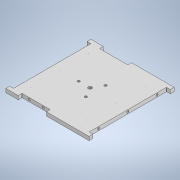
# Autodesk Inventor part: baza
Saved by Autodesk Inventor 2020 (Build 240168000, 168)
## iProperties
Created: 2020-08-17
Part Number: baza
Material: Generic
Document SubType Name: Modeling
Designer: Hesekiel
Density: 1 g/cm^3
Appearance: Default
Author: Hesekiel
Autodesk Inventor part; units mm, degrees
ref_plane "YZ Plane" through (0, 0, 0) normal (1, 0, 0) x (0, 1, 0)
ref_plane "XZ Plane" through (0, 0, 0) normal (0, 1, 0) x (-1, 0, 0)
ref_plane "XY Plane" through (0, 0, 0) normal (0, 0, 1) x (1, 0, 0)
sketch "Sketch1" plane through (0, 0, 0) normal (0, 1, 0) x (-1, 0, 0)
  line L0 (-50, 112.5) -> (50, 112.5)
  line L1 (50, 112.5) -> (50, -112.5)
  line L2 (50, -112.5) -> (-50, -112.5)
  line L3 (-50, -112.5) -> (-50, 112.5)
  line L4 (-50, 112.5) -> (50, -112.5) construction
  line L5 (50, 112.5) -> (-50, -112.5) construction
  line L6 (-37.5, -102.5) -> (37.5, -102.5)
  line L7 (37.5, -102.5) -> (37.5, 102.5)
  line L8 (37.5, 102.5) -> (-37.5, 102.5)
  line L9 (-37.5, 102.5) -> (-37.5, -102.5)
  line L10 (-37.5, -102.5) -> (37.5, 102.5) construction
  line L11 (37.5, -102.5) -> (-37.5, 102.5) construction
  line L12 (37.5, 112.5) -> (37.5, -112.5)
  line L13 (-37.5, 112.5) -> (-37.5, -112.5)
  line L14 (-50, -112.5) -> (-150, -112.5)
  line L15 (-150, 112.5) -> (-50, 112.5)
  line L16 (-50, 112.5) -> (-50, -112.5)
  line L17 (-150, -112.5) -> (-140, -112.5)
  line L18 (-140, -112.5) -> (-140, 112.5)
  line L19 (-150, -112.5) -> (-150, -102.5)
  line L20 (-150, -102.5) -> (-140, -102.5)
  line L21 (-140, 112.5) -> (-140, 102.5)
  line L22 (-140, 102.5) -> (-150, 102.5)
  line L23 (50, 112.5) -> (70, 112.5)
  line L24 (70, -112.5) -> (50, -112.5)
  line L25 (50, -112.5) -> (50, 112.5)
  line L26 (70, -112.5) -> (70, -102.5)
  line L27 (70, 112.5) -> (70, 102.5)
  line L28 (70, -102.5) -> (60, -102.5)
  line L29 (60, -102.5) -> (60, 102.5)
  line L30 (60, 102.5) -> (70, 102.5)
  line L31 (-150, 102.5) -> (-150, 112.5)
  point P0 (0, 0)
  dimension "d0" = 100
  dimension "d2" = 75
  dimension "d3" = 205
  dimension "d49" = 100
  dimension "d50" = 10
  dimension "d51" = 10
  dimension "d52" = 10
  constraints: 64 end point, 11 point on line, 7 parallel, 5 horizontal, 5 perpendicular, 4 midpoint, 1 vertical
  measures "d0" distance of L1.end L2.end
  measures "d2" distance of L8.end L7.end
  measures "d3" distance of L7.end L6.end
  measures "d49" distance of L15.start L15.end
  measures "d50" distance of L14.end L17.end
  measures "d51" distance of L14.end L19.end
  measures "d52" distance of L18.end L21.end
extrude "Extrusion1" add sketch "Sketch1" along normal blind 10 contours L0 L13 L9 L2 L3 | L3 L14 L18 L15 | L18 L22 L31 L15 | L0 L1 L2 L12 L7 | L8 L7 L6 L9 | L14 L19 L20 L18 | L23 L27 L30 L29 L28 L26 L24 L1
sketch "Sketch2" plane through (-37.5, 0, 102.5) normal (0, 0, 1) x (1, 0, 0)
  line L0 (0, 0) -> (75, 0) projected
  line L1 (75, 0) -> (75, 10) projected
  line L2 (0, 10) -> (75, 10) projected
  line L3 (0, 0) -> (0, 10) projected
  line L4 (37.5, 0) -> (37.5, 10)
  line L5 (75, 10) -> (0, 10) projected
  line L6 (37.5, 5) -> (0, 5)
  line L7 (0, 0) -> (0, 10) projected
  line L8 (37.5, 5) -> (75, 5)
  line L9 (75, 0) -> (75, 10) projected
  circle A0 centre (18.75, 5) radius 3
  circle A1 centre (56.25, 5) radius 3
  dimension "d6" = 6
  dimension "d7" = 6
  constraints: 6 end point, 6 midpoint, 2 centre point
  measures "d6" diameter of A0
  measures "d7" diameter of A1
extrude "Extrusion2" cut sketch "Sketch2" against normal blind 20 contours A0 L6 | L6 A0 | A1 L8 | L8 A1
thread "Thread1" size "M6x1" class "6H" standard "ANSI Metric M Profile" full length
thread "Thread2" size "M6x1" class "6H" standard "ANSI Metric M Profile" full length
sketch "Sketch3" plane through (37.5, 0, -102.5) normal (0, 0, -1) x (-1, 0, 0)
  circle A0 centre (18.75, 5) radius 3 projected
  circle A1 centre (56.25, 5) radius 3 projected
  point P0 (37.5, 0)
extrude "Extrusion3" cut sketch "Sketch3" against normal blind 20
thread "Thread3" size "M6x1" class "6H" standard "ANSI Metric M Profile" full length
thread "Thread4" size "M6x1" class "6H" standard "ANSI Metric M Profile" full length
sketch "Sketch4" plane through (-18.75, 5, 82.5) normal (0, 0, 1) x (1, 0, 0)
  point P0 (0, 0)
hole "Hole1" at (-18.75, 5, 82.5) direction (0, 0, -1) diameter 4.917 depth 3 tip angle 120 thread size "M6x1" class "6H" standard "ISO Metric profile"
sketch "Sketch5" plane through (18.75, 5, 82.5) normal (0, 0, 1) x (1, 0, 0)
  point P0 (0, 0)
hole "Hole3" at (18.75, 5, 82.5) direction (0, 0, -1) diameter 4.917 depth 3 tip angle 120 thread size "M6x1" class "6H" standard "ISO Metric profile"
sketch "Sketch6" plane through (18.75, 5, -82.5) normal (0, 0, -1) x (-1, 0, 0)
  point P0 (0, 0)
hole "Hole5" at (18.75, 5, -82.5) direction (0, 0, 1) diameter 4.917 depth 3 tip angle 120 thread size "M6x1" class "6H" standard "ISO Metric profile"
sketch "Sketch7" plane through (-18.75, 5, -82.5) normal (0, 0, -1) x (-1, 0, 0)
  point P0 (0, 0)
hole "Hole7" at (-18.75, 5, -82.5) direction (0, 0, 1) diameter 4.917 depth 3 tip angle 120 thread size "M6x1" class "6H" standard "ISO Metric profile"
fillet "Fillet1" radius 1 6 edges at (-37.5, 5, 102.5) (37.5, 5, 102.5) (-37.5, 5, -102.5) (37.5, 5, -102.5) (140, 5, -102.5) (140, 5, 102.5)
sketch "Sketch8" plane through (140, 0, 101.5) normal (1, 0, 0) x (0, 0, -1)
  line L0 (0, 0) -> (0, 10) projected
  line L1 (0, 0) -> (203, 0) projected
  line L2 (203, 10) -> (203, 0) projected
  line L3 (0, 10) -> (203, 10) projected
  line L4 (214, 10) -> (-11, 10) projected
  circle A0 centre (101.5, 5) radius 3
  line L5 (203, 10) -> (203, 0) projected
  circle A1 centre (179, 5) radius 3
  circle A2 centre (24, 5) radius 3
  line L6 (-1, 0) -> (-1, 10) projected
  line L7 (-1, 5) -> (24, 5)
  line L8 (24, 5) -> (101.5, 5)
  line L9 (204, 0) -> (214, 0) projected
  line L10 (214, 0) -> (214, 10) projected
  line L11 (204, 10) -> (214, 10) projected
  line L12 (204, 0) -> (204, 10) projected
  line L13 (214, 0) -> (214, 10) projected
  line L14 (214, 10) -> (204, 10) projected
  line L15 (204, 0) -> (204, 10) projected
  line L16 (101.5, 5) -> (179, 5)
  point P0 (101.5, 0)
  dimension "d54" = 6
  dimension "d57" = 6
  dimension "d59" = 6
  dimension "d130" = 25
  dimension "d131" = 77.5
  constraints: 6 end point, 3 centre point, 2 perpendicular, 1 horizontal, 1 midpoint
  measures "d54" diameter of A0
  measures "d57" diameter of A1
  measures "d59" diameter of A2
  measures "d130" distance of L7.start L7.end
  measures "d131" distance of L8.end L16.end
extrude "Extrusion4" cut sketch "Sketch8" against normal blind 30 contours L16 L8 A0 | A0 L8 L16 | A1 | L8 L7 A2 | A2 L7 L8
thread "Thread5" size "M6x1" class "6H" standard "ANSI Metric M Profile" full length
thread "Thread6" size "M6x1" class "6H" standard "ANSI Metric M Profile" full length
thread "Thread7" size "M6x1" class "6H" standard "ANSI Metric M Profile" full length
sketch "Sketch12" plane through (-60, 0, -102.5) normal (-1, 0, 0) x (0, 0, 1)
  circle A0 centre (25, 5) radius 3 projected
  circle A1 centre (102.5, 5) radius 3 projected
  circle A2 centre (180, 5) radius 3 projected
  line L0 (204, 0) -> (204, 10) projected
  line L1 (204, 0) -> (1, 0) projected
  line L2 (1, 10) -> (1, 0) projected
  line L3 (204, 10) -> (1, 10) projected
  point P0 (102.5, 0)
extrude "Extrusion5" cut sketch "Sketch12" against normal blind 20 contours A0 | A1 | A2
thread "Thread8" size "M6x1" class "6H" standard "ANSI Metric M Profile" full length
thread "Thread9" size "M6x1" class "6H" standard "ANSI Metric M Profile" full length
thread "Thread10" size "M6x1" class "6H" standard "ANSI Metric M Profile" full length
sketch "Sketch9" plane through (110, 5, 77.5) normal (1, 0, 0) x (0, 0, -1)
  point P0 (-0.375, 0)
sketch "Sketch10" plane through (110, 5, 0) normal (1, 0, 0) x (0, 0, -1)
  point P0 (0, 0)
sketch "Sketch11" plane through (110, 5, -77.5) normal (1, 0, 0) x (0, 0, -1)
  point P0 (0.375, 0)
sketch "Sketch13" plane through (-40, 5, -77.5) normal (-1, 0, 0) x (0, 0, 1)
  point P0 (0.625, 0)
sketch "Sketch14" plane through (-40, 5, 0) normal (-1, 0, 0) x (0, 0, 1)
  point P0 (0, 0)
sketch "Sketch15" plane through (-40, 5, 77.5) normal (-1, 0, 0) x (0, 0, 1)
  point P0 (0.375, 0)
sketch "Sketch16" plane through (110, 5, 77.5) normal (1, 0, 0) x (0, 0, -1)
  point P0 (0, 0)
hole "Hole20" at (110, 5, 77.5) direction (-1, 0, 0) diameter 4.917 depth 3 tip angle 120 thread size "M6x1" class "6H" standard "ISO Metric profile"
sketch "Sketch17" plane through (110, 5, 0) normal (1, 0, 0) x (0, 0, -1)
  point P0 (0, 0)
hole "Hole22" at (110, 5, 0) direction (-1, 0, 0) diameter 4.917 depth 3 tip angle 120 thread size "M6x1" class "6H" standard "ISO Metric profile"
sketch "Sketch18" plane through (110, 5, -77.5) normal (1, 0, 0) x (0, 0, -1)
  point P0 (0, 0)
hole "Hole24" at (110, 5, -77.5) direction (-1, 0, 0) diameter 4.917 depth 3 tip angle 120 thread size "M6x1" class "6H" standard "ISO Metric profile"
sketch "Sketch22" plane through (-40, 5, 77.5) normal (-1, 0, 0) x (0, 0, 1)
  point P0 (0, 0)
hole "Hole31" at (-40, 5, 77.5) direction (1, 0, 0) diameter 4.917 depth 8 tip angle 120 thread size "M6x1" class "6H" standard "ISO Metric profile"
sketch "Sketch23" plane through (-40, 5, 0) normal (-1, 0, 0) x (0, 0, 1)
  point P0 (0, 0)
hole "Hole33" at (-40, 5, 0) direction (1, 0, 0) diameter 4.917 depth 8 tip angle 120 thread size "M6x1" class "6H" standard "ISO Metric profile"
sketch "Sketch24" plane through (-40, 5, -77.5) normal (-1, 0, 0) x (0, 0, 1)
  point P0 (0, 0)
hole "Hole35" at (-40, 5, -77.5) direction (1, 0, 0) diameter 4.917 depth 8 tip angle 120 thread size "M6x1" class "6H" standard "ISO Metric profile"
sketch "Sketch25" plane through (0, 10, 0) normal (0, 1, 0) x (1, 0, 0)
  line L0 (-70, -112.5) -> (-37.5, -112.5) projected
  line L1 (-37.5, -112.5) -> (-37.5, -103.5) projected
  arc A0 (-36.5, -102.5) -> (-37.5, -103.5) centre (-36.5, -103.5) ccw projected
  line L2 (-36.5, -102.5) -> (36.5, -102.5) projected
  arc A1 (37.5, -103.5) -> (36.5, -102.5) centre (36.5, -103.5) ccw projected
  line L3 (37.5, -103.5) -> (37.5, -112.5) projected
  line L4 (37.5, -112.5) -> (150, -112.5) projected
  line L5 (150, -112.5) -> (150, -102.5) projected
  line L6 (150, -102.5) -> (141, -102.5) projected
  arc A2 (140, -101.5) -> (141, -102.5) centre (141, -101.5) ccw projected
  line L7 (140, -101.5) -> (140, 101.5) projected
  arc A3 (141, 102.5) -> (140, 101.5) centre (141, 101.5) ccw projected
  line L8 (141, 102.5) -> (150, 102.5) projected
  line L9 (150, 102.5) -> (150, 112.5) projected
  line L10 (150, 112.5) -> (37.5, 112.5) projected
  line L11 (37.5, 112.5) -> (37.5, 103.5) projected
  arc A4 (36.5, 102.5) -> (37.5, 103.5) centre (36.5, 103.5) ccw projected
  line L12 (36.5, 102.5) -> (-36.5, 102.5) projected
  arc A5 (-37.5, 103.5) -> (-36.5, 102.5) centre (-36.5, 103.5) ccw projected
  line L13 (-37.5, 103.5) -> (-37.5, 112.5) projected
  line L14 (-37.5, 112.5) -> (-70, 112.5) projected
  line L15 (-70, 112.5) -> (-70, 102.5) projected
  line L16 (-70, 102.5) -> (-60, 102.5) projected
  line L17 (-60, 102.5) -> (-60, -102.5) projected
  line L18 (-60, -102.5) -> (-70, -102.5) projected
  line L19 (-70, -102.5) -> (-70, -112.5) projected
  line L20 (140, -101.5) -> (140, 101.5) projected
  line L21 (140, 0) -> (-60, 0)
  line L22 (-60, -3) -> (-60, 3) projected
  line L23 (-70, -112.5) -> (-37.5, -112.5) projected
  line L24 (37.5, -112.5) -> (150, -112.5) projected
  line L25 (-70, -112.5) -> (150, -112.5)
  line L26 (40, -112.5) -> (40, 0)
  circle A6 centre (40, 0) radius 4.765
  circle A7 centre (40, 0) radius 30
  circle A8 centre (10, 0) radius 3.175
  line L27 (40, 0) -> (70, 0) construction
  line L28 (40, 0) -> (53.3501, -23.1231)
  line L29 (53.3501, -23.1231) -> (55, -25.9808)
  circle A9 centre (55, 25.9808) radius 3.175
  circle A10 centre (55, -25.9808) radius 3.175
  line L30 (40, 0) -> (55, 25.9808)
  line L31 (40, 0) -> (70, 0) construction
  line L32 (40, 0) -> (55, -25.9808)
  line L33 (40, 0) -> (70, 0) construction
  point P0 (0, 0)
  dimension "d195" = 9.53
  dimension "d200" = 60
  dimension "d201" = 6.35
  dimension "d203" = 6.35
  dimension "d204" = 6.35
  dimension "d211" = 60
  dimension "d212" = 60
  constraints: 20 end point, 5 centre point, 4 horizontal, 4 midpoint, 4 point on circle, 3 coincident, 2 equal length, 2 point on line
  measures "d195" diameter of A6
  measures "d200" diameter of A7
  measures "d201" diameter of A8
  measures "d203" diameter of A9
  measures "d204" diameter of A10
  measures "d211" angle of L31 L30
  measures "d212" angle of L32 L33
extrude "Extrusion6" cut sketch "Sketch25" against normal up to surface (10 mm away) contours A6 L21 L26 | L26 L28 A6 | A8 L21 A7 | A7 L21 A8 | A10 L29 A7 | A7 A10 | A8 A7 L21 | L30 A6 L21 | L21 A6 L28 | L21 A6 L30 | A7 A8 L21 | L29 A10 A7 | A9 A7 | A7 L30 A9 | L30 A7 A9
thread "Thread14" size "3/8-20 UN" class "2B" standard "ANSI Unified Screw Threads" full length
thread "Thread15" size "1/4-20 UNC" class "2B" standard "ANSI Unified Screw Threads" full length
thread "Thread16" size "1/4-20 UNC" class "2B" standard "ANSI Unified Screw Threads" full length
thread "Thread17" size "1/4-20 UNC" class "2B" standard "ANSI Unified Screw Threads" full length
body "Solid1"
